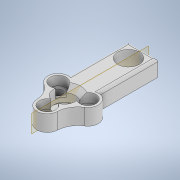
# Autodesk Inventor part: motorholder-nocurvature
Saved by Autodesk Inventor 2020 (Build 240168000, 168)
## iProperties
Created: 2020-03-28
Part Number: motorholder-nocurvature
Material: Generic
Document SubType Name: Modeling
Designer: Adam
Density: 1 g/cm^3
Appearance: Default
Author: Adam
Autodesk Inventor part; units mm, degrees
ref_plane "XZ Plane" through (0, 0, 0) normal (0, 1, 0) x (-1, 0, 0)
ref_plane "XY Plane" through (0, 0, 0) normal (0, 0, 1) x (1, 0, 0)
sketch "Sketch2" plane through (0, 0, 0) normal (0, 1, 0) x (-1, 0, 0)
  line L0 (0, 0) -> (10, 0)
  line L1 (10, 0) -> (10, -20)
  line L2 (10, -20) -> (0, -20)
  line L3 (0, -20) -> (0, 0)
  dimension "d0" = 20
  dimension "d1" = 10
  constraints: 8 end point, 2 parallel, 1 horizontal, 1 perpendicular
  measures "d0" distance of L0.end L1.end
  measures "d1" distance of L1.end L2.end
extrude "Extrusion1" add sketch "Sketch2" along normal blind 3
sketch "Sketch3" plane through (0, 3, 0) normal (0, 1, 0) x (1, 0, 0)
  line L0 (-10, 20) -> (-10, 0) projected
  line L1 (0, 20) -> (-10, 20) projected
  line L2 (-10, 0) -> (0, 0) projected
  circle A0 centre (-5, 2.25) radius 0.8
  circle A1 centre (-5, 2.25) radius 1.5
  circle A2 centre (-5, 5.43) radius 2
  point P0 (-4.2781, 3.5648)
  point P1 (-5.7219, 3.5648)
  dimension "d4" = 5
  dimension "d7" = 0
  dimension "d8" = 3.18
  dimension "d10" = 1.6
  dimension "d11" = 2.25
  dimension "d12" = 3
  dimension "d13" = 4
  constraints: 3 centre point, 3 coincident
  measures "d4" distance from line of L0 point (-5, 5.43)
  measures "d7" horizontal distance of point (-5, 5.43) point (-5, 2.25)
  measures "d8" distance of point (-5, 5.43) point (-5, 2.25)
  measures "d10" diameter of A0
  measures "d11" distance from line of L2 A0.centre
  measures "d12" diameter of A1
  measures "d13" diameter of A2
extrude "Extrusion2" cut sketch "Sketch3" against normal through all contours A0
pattern_circular "Circular Pattern1" count 3 over 360 about axis through (-5, 3, -5.43) along (0, 1, 0) of "Extrusion2"
ref_plane "Work Plane2" through (0, 1.3, 0) normal (0, -1, 0) x (1, 0, 0)
ref_plane "Work Plane1" through (0, 0, 0) normal (0, -1, 0) x (1, 0, 0)
extrude "Extrusion3" cut sketch "Sketch3" against normal up to surface (1.7 mm away) contours A0 | A1 A2 | A2 A1 picked at (-5.474, 3.3061) picked at (-4.9499, 3.5442)
extrude "Extrusion4" cut sketch "Sketch3" against normal through all contours A2 A1 | A1 A2 picked at (-4.9499, 3.5442) picked at (-4.9466, 6.1911)
pattern_circular "Circular Pattern2" count 3 over 360 about axis through (-5, 3, -5.43) along (0, 1, 0) of "Extrusion4", "Extrusion3"
sketch "Sketch6" plane through (0, 3, 0) normal (0, 1, 0) x (1, 0, 0)
  arc A0 (-6.2543, 6.9878) -> (-6.9762, 5.7374) centre (-7.754, 7.02) ccw projected
  circle A1 centre (-7.754, 7.02) radius 1.925
  arc A2 (-3.7457, 6.9878) -> (-6.2543, 6.9878) centre (-5, 5.43) ccw projected
  circle A3 centre (-5, 2.25) radius 1.925
  circle A4 centre (-2.246, 7.02) radius 1.925
  arc A5 (-6.9234, 2.1727) -> (-8.7827, 5.3929) centre (-10.9202, 2.012) ccw
  arc A6 (-1.2173, 5.3929) -> (-3.0766, 2.1727) centre (0.9202, 2.012) ccw
  arc A7 (-6.8592, 8.7244) -> (-3.1408, 8.7244) centre (-5, 12.2661) ccw
  line L0 (-7.754, 8.945) -> (-7.754, 22.7123)
  line L1 (-7.754, 22.7123) -> (-16.28, 22.7123)
  line L2 (-16.28, 22.7123) -> (-16.28, -9.8438)
  line L3 (-16.28, -9.8438) -> (12.2065, -9.8438)
  line L4 (12.2065, -9.8438) -> (12.2065, 22.7123)
  line L5 (12.2065, 22.7123) -> (-2.5928, 22.7123)
  line L6 (-2.246, 8.945) -> (-2.246, 22.7123)
  point P0 (0, 0)
  point P1 (-1.2173, 5.3929)
  point P2 (-3.0766, 2.1727)
  dimension "d35" = 0.425
  dimension "d38" = 360
  dimension "d40" = 4
  dimension "d43" = 360
  constraints: 14 end point, 8 point on circle, 4 centre point, 4 perpendicular, 3 point on line, 2 vertical, 1 coincident, 1 tangent, 27 other
  measures "d35" radial gap between concentric circles of A1 A0
  measures "d40" radius of A5
extrude "Extrusion5" cut sketch "Sketch6" against normal through all contours A1 A5 A3 A6 A4 L6 L5 L4 L3 L2 L1 L0
sketch "Sketch7" plane through (0, 3, 0) normal (0, 1, 0) x (1, 0, 0)
  point P0 (0, 0)
  point P1 (-5.0309, 17.3385)
hole "Hole1" at (-5.0309, 3, -17.3385) direction (0, -1, 0) diameter 4 end through all
chamfer "Chamfer1" distance 1 angle 45 1 edges at (-5, 3, -7.43)
chamfer "Chamfer2" distance 0.5 angle 45 1 edges at (-4.2781, 0, -7.2952)
ref_plane "Work Plane3" through (-5, 0, -1.45) normal (1, 0, 0) x (0, 1, 0)
fillet "Fillet4" radius 0.5 3 edges at (-5, 3, -20) (-2.246, 3, -14.4725) (-7.754, 3, -14.4725)
equation "\"d4\" = 0.5 * d1"
body "Solid1"
